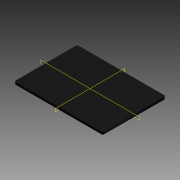
# Autodesk Inventor part: D-052
Saved by Autodesk Inventor 2015 (Build 190159000, 159)
## iProperties
Company: MARCHA TECHNOLOGY
Created: 2014-02-26
Part Number: D-052
Document SubType Name: Modeling
Designer: O.Martin
Density: 1 g/cm^3
Project: WITBOXprinter_V04
Description: CRISTAL
Stock Number: 28001
Mass: 532.942 g
Surface Area: 1434.03 cm^2
Volume: 532.942 cm^3
Material: Generic
Appearance: Black Vinyl (texture)
Author: O.Martin
Autodesk Inventor part; units mm, degrees
ref_plane "XY Plane" through (0, 0, 0) normal (0, 0, 1) x (1, 0, 0)
sketch "Boceto1" plane through (0, 0, 0) normal (0, 0, 1) x (1, 0, 0)
  line L0 (152.65, -108.5) -> (-152.65, -108.5)
  line L1 (-152.65, -108.5) -> (-152.65, 108.5)
  line L2 (-152.65, 108.5) -> (152.65, 108.5)
  line L3 (152.65, 108.5) -> (152.65, -108.5)
  point P0 (0, 0)
  point P1 (152.65, 0)
  point P2 (0, -108.5)
  dimension "d0" = 305.3
  dimension "d1" = 217
  constraints: 8 end point, 2 midpoint, 2 parallel, 1 horizontal, 1 horizontal alignment, 1 perpendicular, 1 vertical alignment
  measures "d0" distance of L1.end L2.end
  measures "d1" distance of L0.end L1.end
extrude "Extrusión1" add sketch "Boceto1" along normal blind 8
fillet "Empalme1" radius 5 4 edges at (-152.65, 108.5, 4) (-152.65, -108.5, 4) (152.65, -108.5, 4) (152.65, 108.5, 4)
sketch "Boceto2" plane through (0, 0, 8) normal (0, 0, 1) x (1, 0, 0)
  line L0 (-148.5, 105) -> (148.5, 105)
  line L1 (148.5, 105) -> (148.5, -105)
  line L2 (148.5, -105) -> (-148.5, -105)
  line L3 (-148.5, -105) -> (-148.5, 105)
  line L4 (-147.65, 108.5) -> (147.65, 108.5) projected
  line L5 (-152.65, -103.5) -> (-152.65, 103.5) projected
  point P0 (-148.5, 0)
  point P1 (-154.5, 0)
  point P2 (0, -105)
  point P3 (0, -109.5)
  point P4 (-152.65, 0)
  point P5 (0, 105)
  point P6 (0, 108.5)
  dimension "d11" = 297
  dimension "d12" = 210
  constraints: 8 end point, 5 midpoint, 2 horizontal alignment, 2 parallel, 2 vertical alignment, 1 horizontal, 1 perpendicular
  measures "d11" distance of L1.end L2.end
  measures "d12" distance of L2.end L0.start
extrude "Limites" cut sketch "Boceto2" against normal blind 0.1
sketch "Boceto3" plane through (0, 0, 0) normal (0, 0, -1) x (-1, 0, 0)
  line L0 (-147.65, -108.5) -> (147.65, -108.5) projected
  line L1 (147.65, 108.5) -> (-147.65, 108.5) projected
  line L2 (65.1, -108.5) -> (-65.1, -108.5)
  line L3 (-65.1, -108.5) -> (-65.1, -107.5)
  line L4 (-65.1, -107.5) -> (65.1, -107.5)
  line L5 (65.1, -107.5) -> (65.1, -108.5)
  line L6 (65.1, 108.5) -> (-65.1, 108.5)
  line L7 (-65.1, 108.5) -> (-65.1, 107.5)
  line L8 (-65.1, 107.5) -> (65.1, 107.5)
  line L9 (65.1, 107.5) -> (65.1, 108.5)
  point P0 (0, -108.5)
  point P1 (0, 108.5)
  dimension "d15" = 130.2
  dimension "d16" = 215
  constraints: 16 end point, 4 midpoint, 4 parallel, 2 equal length, 2 horizontal, 2 perpendicular, 2 point on line
  measures "d15" distance of L7.end L8.end
  measures "d16" distance between parallel lines of L4 L8
extrude "Extrusión3" [suppressed]
sketch "POSICION IMANES" plane through (0, 0, 0) normal (0, 0, -1) x (-1, 0, 0)
  line L0 (-147.65, -108.5) -> (147.65, -108.5)
  line L1 (152.65, -103.5) -> (152.65, 103.5)
  line L2 (52.5, -93.5) -> (-52.5, -93.5) construction
  line L3 (-52.5, -93.5) -> (-52.5, 93.5) construction
  line L4 (-52.5, 93.5) -> (52.5, 93.5) construction
  line L5 (52.5, 93.5) -> (52.5, -93.5) construction
  line L6 (152.65, -103.5) -> (152.65, 103.5) construction
  line L7 (-152.65, 103.5) -> (-152.65, -103.5) construction
  circle A0 centre (-52.5, 93.5) radius 10
  circle A1 centre (52.5, 93.5) radius 10
  circle A2 centre (52.5, -93.5) radius 10
  circle A3 centre (-52.5, -93.5) radius 10
  arc A4 (-147.65, 108.5) -> (-152.65, 103.5) centre (-147.65, 103.5) ccw projected
  line L8 (-152.65, 103.5) -> (-152.65, -103.5) projected
  arc A5 (-152.65, -103.5) -> (-147.65, -108.5) centre (-147.65, -103.5) ccw projected
  line L9 (-147.65, -108.5) -> (147.65, -108.5) projected
  arc A6 (147.65, -108.5) -> (152.65, -103.5) centre (147.65, -103.5) ccw projected
  line L10 (152.65, -103.5) -> (152.65, 103.5) projected
  arc A7 (152.65, 103.5) -> (147.65, 108.5) centre (147.65, 103.5) ccw projected
  line L11 (147.65, 108.5) -> (-147.65, 108.5) projected
  point P0 (0, -93.5)
  point P1 (52.5, 0)
  point P2 (152.65, 0)
  point P3 (0, -108.5)
  dimension "d19" = 15
  dimension "d21" = 20
  dimension "d22" = 105
  constraints: 16 end point, 4 centre point, 4 coincident, 4 midpoint, 3 equal radius, 2 parallel, 1 horizontal, 1 horizontal alignment, 1 perpendicular, 1 vertical alignment
  measures "d19" distance between parallel lines of L0 L2
  measures "d21" diameter of A2
  measures "d22" distance of L2.start L2.end
sketch "Boceto5" plane through (0, 0, 0) normal (0, 0, -1) x (-1, 0, 0)
  line L0 (-152.65, 103.5) -> (-152.65, -103.5) projected
  line L1 (-147.65, -108.5) -> (147.65, -108.5) projected
  circle A0 centre (0, -98.5) radius 2
  point P0 (-152.65, 0)
  point P1 (0, 0)
  point P2 (0, -108.5)
  point P3 (0, -108.5)
  point P4 (0, -108.5)
  dimension "d28" = 4
  dimension "d29" = 98.5
  constraints: 4 midpoint, 2 vertical alignment, 1 centre point, 1 horizontal alignment
  measures "d28" diameter of A0
  measures "d29" distance of A0.centre point (0, 0)
body "Solid1"
